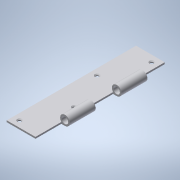
# Autodesk Inventor part: Part2
Saved by Autodesk Inventor 2020.2 (Build 242310000, 310)
## iProperties
Created: 2013-11-30
Part Number: Part2
Material: Generic
Document SubType Name: Modeling
Designer: NiveshandNisheeth
Density: 1 g/cm^3
Appearance: Cool White
Author: NiveshandNisheeth
Autodesk Inventor part; units mm, degrees
ref_plane "YZ Plane" through (0, 0, 0) normal (1, 0, 0) x (0, 1, 0)
ref_plane "XZ Plane" through (0, 0, 0) normal (0, 1, 0) x (-1, 0, 0)
sketch "Sketch1" plane through (0, 0, 0) normal (0, 0, 1) x (1, 0, 0)
  line L0 (0, 0) -> (-31.75, 0)
  line L1 (-31.75, 0) -> (-31.75, 1.5875)
  line L2 (-31.75, 1.5875) -> (0, 1.5875)
  line L3 (0, 1.5875) -> (0, 0)
  circle A0 centre (0, 4.7625) radius 4.7625
  circle A1 centre (0, 4.7625) radius 3.175
  dimension "d0" = 31.75
  dimension "d1" = 1.5875
  dimension "d2" = 9.525
  dimension "d3" = 6.35
  constraints: 8 end point, 2 centre point, 2 parallel, 1 coincident, 1 horizontal, 1 perpendicular, 1 tangent, 1 vertical alignment
  measures "d0" distance of L1.end L2.end
  measures "d1" distance of L0.end L1.end
  measures "d2" diameter of A0
  measures "d3" diameter of A1
extrude "Extrusion1" add sketch "Sketch1" along normal mid plane 127
ref_plane "Work Plane1" through (0, 0, 38.1) normal (0, 0, 1) x (1, 0, 0)
sketch "Sketch2" plane through (0, 0, 38.1) normal (0, 0, 1) x (1, 0, 0)
  arc A0 (0, 0) -> (-3.5498, 1.5875) centre (0, 4.7625) ccw projected
  line L0 (-3.5498, 1.5875) -> (-3.5498, 0)
  line L1 (-3.5498, 0) -> (0, 0)
  constraints: 4 end point, 1 perpendicular, 1 tangent, 1 vertical
extrude "Extrusion2" cut sketch "Sketch2" along normal blind 25.4
pattern_linear "Rectangular Pattern1" count 3 spacing 50.8 along (0, 0, -1) of "Extrusion2"
sketch "Sketch3" plane through (-31.75, 1.5875, -63.5) normal (0, 1, 0) x (1, 0, 0)
  line L0 (28.2002, 0) -> (0, 0) construction
  line L1 (0, -127) -> (28.2002, -127) construction
  line L2 (0, 0) -> (28.2002, 0) construction
  line L3 (28.2002, 0) -> (28.2002, -127) construction
  line L4 (28.2002, -127) -> (0, -127) construction
  line L5 (0, -127) -> (0, 0) construction
  line L6 (21.8502, -120.65) -> (21.8502, -6.35) construction
  line L7 (21.8502, -6.35) -> (6.35, -6.35) construction
  line L8 (6.35, -6.35) -> (6.35, -120.65) construction
  line L9 (6.35, -120.65) -> (21.8502, -120.65) construction
  line L10 (6.35, -82.55) -> (21.8502, -82.55) construction
  line L11 (6.35, -44.45) -> (21.8502, -44.45) construction
  line L12 (6.35, -6.35) -> (21.8502, -6.35) construction
  point P0 (31.75, -63.5)
  dimension "d12" = 6.35
  dimension "d15" = 114.3
  constraints: 22 end point, 4 parallel, 2 perpendicular, 1 horizontal, 1 vertical, 12 other
  measures "d12" distance between parallel lines of L8 L5
  measures "d15" distance of L8.end L12.start
hole "Hole1" at (-9.8998, 1.5875, -57.15) at (-25.4, 1.5875, 57.15) at (-9.8998, 1.5875, 19.05) at (-25.4, 1.5875, -19.05) direction (0, -1, 0) diameter 3.175 end through all
chamfer "Chamfer1" distance 0.7937 angle 45 4 edges at (-25.4, 1.5875, 55.5625) (-9.8998, 1.5875, 17.4625) (-25.4, 1.5875, -20.6375) (-9.8998, 1.5875, -58.7375)
body "Solid1"
